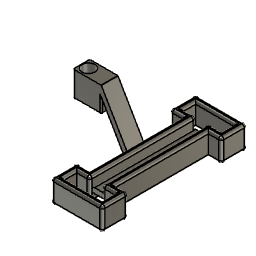
UAS_Legs v1 (Autodesk Fusion 360 design; units mm, degrees)
Autodesk Fusion 360 part; units mm, degrees
sketch "Sketch1" plane through (0, 0, 0) normal (0, 1, 0) x (1, 0, 0)
  line L0 (-3.2108, -13) -> (7.7892, -13)
  line L1 (7.7892, -8) -> (7.7892, -3)
  line L2 (7.7892, -3) -> (-3.2108, -3)
  line L3 (-3.2108, -3) -> (-3.2108, -13)
  line L4 (18.1815, 3) -> (28.1815, 3)
  line L5 (28.1815, 3) -> (28.1815, 12)
  line L6 (28.1815, 12) -> (18.1815, 12)
  line L7 (7.7892, -13) -> (18.1815, 5)
  line L8 (7.7892, -8) -> (18.1815, 10)
  line L9 (18.1815, 12) -> (18.1815, 10)
  line L10 (18.1815, 5) -> (18.1815, 3)
  dimension "d1" = 25
  dimension "d2" = 11
  dimension "d3" = 11
  dimension "d4" = 10
  dimension "d5" = 5
  dimension "d6" = 2
  dimension "d7" = 2
  dimension "d8" = 30
  dimension "d9" = 60
  dimension "d10" = 10
  dimension "d11" = 5
  dimension "d12" = 5
  dimension "d13" = 20.3923
  constraint horizontal L0
  constraint vertical L1
  constraint horizontal L2
  constraint vertical L3
  constraint horizontal L4
  constraint vertical L5
  constraint horizontal L6
  constraint vertical L9
  constraint coincident L7.end L9
  constraint parallel L7 L8
  constraint collinear L9 L10
  measures "d1" vertical distance of L0.start L6.end
  measures "d2" distance of L0.start L0.end
  measures "d3" distance of L1.end L2.end
  measures "d4" distance of L0.start L2.end
  measures "d5" distance of L1.end L1.start
  measures "d6" distance of L6.end L8.end
  measures "d7" distance of L4.start L7.end
  measures "d8" angle of L1 L8
  measures "d9" angle of L0 L7
  measures "d10" distance of L4.start L4.end
  measures "d11" distance of L0.end L1.start
  measures "d12" distance of L7.end L8.end
  measures "d13" horizontal distance of L0.end L4.end
extrude "Extrude1" add sketch "Sketch1" along normal blind 6.5 makes body 1
sketch "Sketch2" plane through (0, 0, 0) normal (0, -1, 0) x (1, 0, 0)
  line L0 (7.7892, 3) -> (7.7892, 8)
  line L1 (7.7892, 8) -> (18.1815, -10)
  line L2 (18.1815, -10) -> (18.1815, -12)
  line L3 (18.1815, -12) -> (28.1815, -12)
  line L4 (28.1815, -12) -> (28.1815, -3)
  line L5 (28.1815, -3) -> (18.1815, -3)
  line L6 (18.1815, -3) -> (18.1815, -5)
  line L7 (18.1815, -5) -> (7.7892, 13)
  line L8 (7.7892, 13) -> (-3.2108, 13)
  line L9 (-3.2108, 13) -> (-3.2108, 3)
  line L10 (-3.2108, 3) -> (7.7892, 3)
  line L11 (18.1815, -3) -> (28.1815, -3)
  line L12 (28.1815, -3) -> (28.1815, -12)
  line L13 (28.1815, -12) -> (18.1815, -12)
  line L14 (18.1815, -12) -> (18.1815, -3)
  constraint horizontal L11
  constraint vertical L12
  constraint horizontal L13
  constraint vertical L14
  constraint coincident L3.end L4.start
  constraint coincident L5.end L6.start
extrude "Extrude2" add sketch "Sketch2" along normal blind 25 contours L2 L3 L4 L5 L6 L11 L12 L13 L14 bodies 1
sketch "Sketch3" plane through (0, 6.5, 0) normal (0, 1, 0) x (-1, 0, 0)
  line L0 (-7.7892, 8) -> (-7.7892, 3)
  line L1 (-7.7892, 3) -> (3.2108, 3)
  line L2 (3.2108, 3) -> (3.2108, 13)
  line L3 (3.2108, 13) -> (-7.7892, 13)
  line L4 (-7.7892, 13) -> (-18.1815, -5)
  line L5 (-18.1815, -5) -> (-18.1815, -3)
  line L6 (-18.1815, -3) -> (-28.1815, -3)
  line L7 (-28.1815, -3) -> (-28.1815, -12)
  line L8 (-28.1815, -12) -> (-18.1815, -12)
  line L9 (-18.1815, -12) -> (-18.1815, -10)
  line L10 (-18.1815, -10) -> (-7.7892, 8)
  line L11 (-28.1815, -3) -> (-18.1815, -3)
  line L12 (-18.1815, -3) -> (-18.1815, -12)
  line L13 (-18.1815, -12) -> (-28.1815, -12)
  line L14 (-28.1815, -12) -> (-28.1815, -3)
  constraint horizontal L11
  constraint vertical L12
  constraint horizontal L13
  constraint vertical L14
  constraint coincident L8.end L9.start
  constraint coincident L6.end L7.start
extrude "Extrude3" add sketch "Sketch3" along normal blind 25 contours L5 L6 L7 L8 L9 L11 L12 L13 L14 bodies 1
sketch "Sketch4" plane through (0, 0, 13) normal (0, 0, 1) x (-1, 0, 0)
  line L0 (3.2108, 0) -> (-7.7892, 0)
  line L1 (-7.7892, 0) -> (-7.7892, -6.5)
  line L2 (-7.7892, -6.5) -> (3.2108, -6.5)
  line L3 (3.2108, -6.5) -> (3.2108, 0)
  circle A0 centre (0.4608, -3.25) radius 2.55
  dimension "d20" = 5.1
  dimension "d21" = 2.75
  dimension "d22" = 3.25
  dimension "d23" = 3
  measures "d20" diameter of A0
  measures "d21" distance of L3 A0.centre
  measures "d22" distance of L2 A0.centre
extrude "Extrude4" cut sketch "Sketch4" against normal blind 10 contours A0 bodies 1
sketch "Sketch5" plane through (18.1815, 0, 0) normal (-1, 0, 0) x (0, -1, 0)
  line L0 (-6.5, -5) -> (0, -5)
  line L1 (0, -5) -> (0, -10)
  line L2 (0, -10) -> (-6.5, -10)
  line L3 (-6.5, -10) -> (-6.5, -5)
  line L4 (25, -3) -> (-31.5, -3)
  line L5 (-31.5, -3) -> (-31.5, -12)
  line L6 (-31.5, -12) -> (25, -12)
  line L7 (25, -12) -> (25, -3)
  line L8 (25, -3) -> (15, -3)
  line L9 (15, -3) -> (15, -12)
  line L10 (15, -12) -> (25, -12)
  line L11 (25, -12) -> (25, -3)
  dimension "d26" = 10
  dimension "d27" = 9
  constraint horizontal L8
  constraint vertical L9
  constraint horizontal L10
  constraint vertical L11
  constraint coincident L6 L9.end
  constraint coincident L4.start L7.end
  measures "d26" distance of L4.start L8.end
  measures "d27" distance of L4.start L6.end
extrude "Extrude5" add sketch "Sketch5" along normal blind 5 contours L4 L6 L7 L8 L9 L10 L11 bodies 1
sketch "Sketch6" plane through (18.1815, 0, 0) normal (-1, 0, 0) x (0, -1, 0)
  line L0 (15, -12) -> (15, -3)
  line L1 (15, -3) -> (-31.5, -3)
  line L2 (-31.5, -3) -> (-31.5, -12)
  line L3 (-31.5, -12) -> (15, -12)
  line L4 (-6.5, -5) -> (0, -5)
  line L5 (0, -5) -> (0, -10)
  line L6 (0, -10) -> (-6.5, -10)
  line L7 (-6.5, -10) -> (-6.5, -5)
  line L8 (-31.5, -3) -> (-21.5, -3)
  line L9 (-21.5, -3) -> (-21.5, -12)
  line L10 (-21.5, -12) -> (-31.5, -12)
  line L11 (-31.5, -12) -> (-31.5, -3)
  dimension "d30" = 10
  dimension "d31" = 9
  constraint horizontal L8
  constraint vertical L9
  constraint horizontal L10
  constraint vertical L11
  constraint coincident L3 L9.end
  constraint coincident L1.end L2.start
  measures "d30" distance of L1.end L8.end
  measures "d31" distance of L1.end L2.end
extrude "Extrude6" add sketch "Sketch6" along normal blind 5 contours L1 L2 L3 L8 L9 L10 L11 bodies 1
sketch "Sketch7" plane through (28.1815, 0, 0) normal (1, 0, 0) x (0, 1, 0)
  line L0 (-25, -12) -> (31.5, -12)
  line L1 (31.5, -12) -> (31.5, -3)
  line L2 (31.5, -3) -> (-25, -3)
  line L3 (-25, -3) -> (-25, -12)
  line L4 (-25, -3) -> (-15, -3)
  line L5 (-15, -3) -> (-15, -12)
  line L6 (-15, -12) -> (-25, -12)
  line L7 (-25, -12) -> (-25, -3)
  dimension "d34" = 10
  dimension "d35" = 9
  constraint horizontal L4
  constraint vertical L5
  constraint horizontal L6
  constraint vertical L7
  constraint coincident L0 L5.end
  constraint coincident L2.end L3.start
  measures "d34" distance of L2.end L4.end
  measures "d35" distance of L2.end L0.start
extrude "Extrude7" add sketch "Sketch7" along normal blind 5 contours L0 L2 L3 L4 L5 L6 L7 bodies 1
sketch "Sketch8" plane through (28.1815, 0, 0) normal (1, 0, 0) x (0, 1, 0)
  line L0 (-15, -3) -> (-15, -12)
  line L1 (-15, -12) -> (31.5, -12)
  line L2 (31.5, -12) -> (31.5, -3)
  line L3 (31.5, -3) -> (-15, -3)
  line L4 (31.5, -3) -> (21.5, -3)
  line L5 (21.5, -3) -> (21.5, -12)
  line L6 (21.5, -12) -> (31.5, -12)
  line L7 (31.5, -12) -> (31.5, -3)
  dimension "d38" = 10
  dimension "d39" = 9
  constraint horizontal L4
  constraint vertical L5
  constraint horizontal L6
  constraint vertical L7
  constraint coincident L1 L5.end
  constraint coincident L2.end L3.start
  measures "d38" distance of L2.end L4.end
  measures "d39" distance of L2.end L1.end
extrude "Extrude8" add sketch "Sketch8" along normal blind 5 contours L1 L2 L3 L4 L5 L6 L7 bodies 1
sketch "Sketch9" plane through (0, 0, -3) normal (0, 0, 1) x (-1, 0, 0)
  line L0 (-28.1815, 15) -> (-28.1815, -21.5)
  line L1 (-28.1815, -21.5) -> (-33.1815, -21.5)
  line L2 (-33.1815, -21.5) -> (-33.1815, -31.5)
  line L3 (-33.1815, -31.5) -> (-13.1815, -31.5)
  line L4 (-13.1815, -31.5) -> (-13.1815, -21.5)
  line L5 (-13.1815, -21.5) -> (-18.1815, -21.5)
  line L6 (-18.1815, -21.5) -> (-18.1815, 15)
  line L7 (-18.1815, 15) -> (-13.1815, 15)
  line L8 (-13.1815, 15) -> (-13.1815, 25)
  line L9 (-13.1815, 25) -> (-33.1815, 25)
  line L10 (-33.1815, 25) -> (-33.1815, 15)
  line L11 (-33.1815, 15) -> (-28.1815, 15)
  line L12 (-15.6815, -29) -> (-30.6815, -29)
  line L13 (-30.6815, -29) -> (-30.6815, -24)
  line L14 (-15.6815, -24) -> (-15.6815, -29)
  line L15 (-25.6815, -24) -> (-25.6815, 17.5)
  line L16 (-20.6815, 17.5) -> (-20.6815, -24)
  line L17 (-30.6815, 17.5) -> (-30.6815, 22.5)
  line L18 (-30.6815, 22.5) -> (-15.6815, 22.5)
  line L19 (-15.6815, 22.5) -> (-15.6815, 17.5)
  line L20 (-30.6815, -24) -> (-25.6815, -24)
  line L21 (-20.6815, -24) -> (-15.6815, -24)
  line L22 (-15.6815, 17.5) -> (-20.6815, 17.5)
  line L23 (-25.6815, 17.5) -> (-30.6815, 17.5)
  dimension "d42" = 2.5
  dimension "d43" = 2.5
  dimension "d44" = 2.5
  dimension "d45" = 5
  dimension "d46" = 2.5
  dimension "d47" = 2.5
  dimension "d48" = 2.5
  dimension "d49" = 2.5
  dimension "d50" = 2.5
  dimension "d51" = 2.5
  dimension "d52" = 2.5
  dimension "d53" = 2.5
  constraint horizontal L12
  constraint vertical L13
  constraint horizontal L20
  constraint vertical L14
  constraint vertical L15
  constraint vertical L16
  constraint coincident L16.end L20
  constraint horizontal L22
  constraint vertical L17
  constraint horizontal L18
  constraint vertical L19
  constraint collinear L20 L21
  constraint collinear L22 L23
  measures "d42" distance of L3 L12
  measures "d43" distance of L2 L13
  measures "d44" distance of L1 L20
  measures "d45" distance of L12.start L14.start
  measures "d46" distance of L4 L14
  measures "d47" distance of L5 L21
  measures "d48" distance of L6 L16
  measures "d49" distance of L0 L15
  measures "d50" distance of L11 L23
  measures "d51" distance of L10 L17
  measures "d52" distance of L9 L18
  measures "d53" distance of L8 L19
extrude "Extrude9" cut sketch "Sketch9" against normal blind 9 contours L12 L13 L14 L15 L16 L17 L18 L19 L20 L21 L22 L23 bodies 1
sketch "Sketch10" plane through (20.6815, 0, 0) normal (1, 0, 0) x (0, 1, 0)
  line L0 (24, -3) -> (-17.5, -3)
  line L1 (-17.5, -3) -> (-17.5, -12)
  line L2 (-17.5, -12) -> (24, -12)
  line L3 (24, -12) -> (24, -3)
  line L4 (-16.5, -6.5) -> (23, -6.5)
  line L5 (23, -6.5) -> (23, -8.5)
  line L6 (23, -8.5) -> (-16.5, -8.5)
  line L7 (-16.5, -8.5) -> (-16.5, -6.5)
  dimension "d56" = 3.5
  dimension "d57" = 3.5
  dimension "d58" = 2
  dimension "d61" = 1
  dimension "d63" = 39.5
  dimension "d64" = 1
  constraint horizontal L4
  constraint vertical L5
  constraint horizontal L6
  constraint vertical L7
  measures "d56" distance of L0 L4
  measures "d57" distance of L2 L6
  measures "d58" distance of L4 L6
  measures "d61" distance of L1 L7
  measures "d63" distance of L4.start L4.end
  measures "d64" distance of L3 L5
extrude "Extrude10" add sketch "Sketch10" along normal blind 5 separate body contours L4 L5 L6 L7 makes body 2
fillet "Fillet1" radius 1 1 edges at (18.1815, 3.25, -3) on bodies 1
fillet "Fillet2" radius 1 1 edges at (20.6815, 3.25, -3) on bodies 1
fillet "Fillet3" radius 1 3 edges at (17.6815, -17.5, -3) (20.3886, -17.5, -3.2929) (20.6815, -17.5, -8) on bodies 1
fillet "Fillet4" radius 1 1 edges at (15.6815, -19.5, -3) on bodies 1
fillet "Fillet5" radius 1 1 edges at (22.6815, -22.5, -3) on bodies 1
fillet "Fillet6" radius 1 1 edges at (30.6815, -20.5, -3) on bodies 1
fillet "Fillet7" radius 1 1 edges at (28.6815, -17.5, -3) on bodies 1
fillet "Fillet8" radius 1 3 edges at (25.6815, 3.75, -3) (25.6815, -17.2071, -3.2929) (25.6815, -17.5, -8) on bodies 1
fillet "Fillet9" radius 1 3 edges at (20.6815, 24, -8) (20.3886, 24, -3.2929) (17.6815, 24, -3) on bodies 1
fillet "Fillet10" radius 1 1 edges at (15.6815, 26, -3) on bodies 1
fillet "Fillet11" radius 1 1 edges at (22.6815, 29, -3) on bodies 1
fillet "Fillet12" radius 1 3 edges at (28.6815, 24, -3) (25.9744, 24, -3.2929) (25.6815, 24, -8) on bodies 1
fillet "Fillet13" radius 1 1 edges at (30.6815, 26.5, -3) on bodies 1
fillet "Fillet14" radius 1 1 edges at (28.1815, 3.25, -3) on bodies 1
fillet "Fillet15" radius 1 1 edges at (30.1815, -15, -3) on bodies 1
fillet "Fillet16" radius 1 3 edges at (33.1815, -15, -8) (33.1815, -15.2929, -3.2929) (33.1815, -20.5, -3) on bodies 1
fillet "Fillet17" radius 1 3 edges at (22.6815, -25, -3) (32.8886, -25, -3.2929) (33.1815, -25, -8) on bodies 1
fillet "Fillet18" radius 1 3 edges at (13.1815, -25, -8) (13.1815, -24.7071, -3.2929) (13.1815, -19.5, -3) on bodies 1
fillet "Fillet19" radius 1 1 edges at (30.1815, 21.5, -3) on bodies 1
fillet "Fillet20" radius 1 3 edges at (33.1815, 27, -3) (33.1815, 21.7929, -3.2929) (33.1815, 21.5, -8) on bodies 1
fillet "Fillet21" radius 1 3 edges at (33.1815, 31.5, -8) (32.8886, 31.5, -3.2929) (22.6815, 31.5, -3) on bodies 1
fillet "Fillet22" radius 1 3 edges at (13.1815, 26, -3) (13.1815, 31.2071, -3.2929) (13.1815, 31.5, -8) on bodies 1
fillet "Fillet23" radius 1 3 edges at (16.6815, 21.5, -3) (13.4744, 21.5, -3.2929) (13.1815, 21.5, -8) on bodies 1
fillet "Fillet24" radius 1 3 edges at (16.6815, -15, -3) (13.4744, -15, -3.2929) (13.1815, -15, -8) on bodies 1
fillet "Fillet25" radius 1 1 edges at (18.1815, 3.25, -12) on bodies 1
fillet "Fillet26" radius 1 9 edges at (30.1815, 21.5, -12) (32.8886, 21.7929, -12) (33.1815, 26.5, -12) (32.8886, 31.2071, -12) (23.1815, 31.5, -12) (13.4744, 31.2071, -12) (13.1815, 26.5, -12) (13.4744, 21.7929, -12) (16.6815, 21.5, -12) on bodies 1
fillet "Fillet27" radius 1 9 edges at (16.6815, -15, -12) (13.4744, -15.2929, -12) (13.1815, -20, -12) (13.4744, -24.7071, -12) (23.1815, -25, -12) (32.8886, -24.7071, -12) (33.1815, -20, -12) (32.8886, -15.2929, -12) (30.1815, -15, -12) on bodies 1
fillet "Fillet28" radius 1 5 edges at (28.6815, -17.5, -12) (25.9744, -17.2071, -12) (25.6815, 3.25, -12) (25.9744, 23.7071, -12) (28.6815, 24, -12) on bodies 1
fillet "Fillet29" radius 1 1 edges at (28.1815, 3.25, -12) on bodies 1
fillet "Fillet30" radius 1 1 edges at (30.6815, 26, -12) on bodies 1
fillet "Fillet31" radius 1 1 edges at (23.6815, 29, -12) on bodies 1
fillet "Fillet32" radius 1 1 edges at (15.6815, 27, -12) on bodies 1
fillet "Fillet33" radius 1 5 edges at (17.1815, 24, -12) (20.3886, 23.7071, -12) (20.6815, 3.25, -12) (20.3886, -17.2071, -12) (17.6815, -17.5, -12) on bodies 1
fillet "Fillet34" radius 1 1 edges at (15.6815, -19.5, -12) on bodies 1
fillet "Fillet35" radius 1 1 edges at (22.6815, -22.5, -12) on bodies 1
fillet "Fillet36" radius 1 1 edges at (30.6815, -20, -12) on bodies 1
fillet "Fillet37" radius 1 1 edges at (25.6815, 3.25, -6.5) on bodies 2
fillet "Fillet38" radius 1 1 edges at (20.6815, 3.25, -6.5) on bodies 2
fillet "Fillet39" radius 0.5 1 edges at (12.9853, 0, -1) on bodies 1
fillet "Fillet40" radius 0.5 1 edges at (2.2892, 0, 3) on bodies 1
fillet "Fillet41" radius 0.5 3 edges at (7.7892, 0, 6.25) (7.7892, 0.1464, 3.1464) (7.7892, 3.5, 3) on bodies 1
fillet "Fillet42" radius 0.5 3 edges at (-3.2108, 3.5, 3) (-3.2108, 0.1464, 3.1464) (-3.2108, 0, 8.25) on bodies 1
fillet "Fillet43" radius 0.5 5 edges at (7.7892, 6.5, 5.75) (7.6427, 6.5, 3.1464) (2.2892, 6.5, 3) (-3.0644, 6.5, 3.1464) (-3.2108, 6.5, 8.25) on bodies 1
fillet "Fillet44" radius 0.5 1 edges at (12.7353, 6.5, -0.567) on bodies 1
fillet "Fillet45" radius 0.5 5 edges at (18.1815, 6.5, -7) (18.1815, 6.3536, -9.7071) (18.1815, 3.25, -10) (18.1815, 0.1464, -9.7071) (18.1815, 0, -7) on bodies 1
fillet "Fillet46" radius 0.1 1 edges at (7.7892, 3.25, 13) on bodies 1
